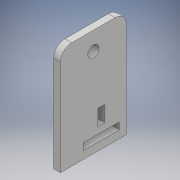
# Autodesk Inventor part: muñeca4
Saved by Autodesk Inventor 2018 (Build 220112000, 112)
## iProperties
Created: 2020-03-11
Part Number: muñeca4
Material: Genérico
Document SubType Name: Modeling
Designer: david
Density: 1 g/cm^3
Appearance: Valor por defecto
Author: david
Autodesk Inventor part; units mm, degrees
ref_plane "YZ Plane" through (0, 0, 0) normal (1, 0, 0) x (0, 1, 0)
ref_plane "XZ Plane" through (0, 0, 0) normal (0, 1, 0) x (-1, 0, 0)
ref_plane "XY Plane" through (0, 0, 0) normal (0, 0, 1) x (1, 0, 0)
sketch "Boceto1" plane through (0, 0, 0) normal (1, 0, 0) x (0, 1, 0)
  line L0 (8, 0) -> (8, -3)
  line L1 (8, -3) -> (-8, -3)
  line L2 (-8, -3) -> (-8, 0)
  line L3 (8, 0) -> (-8, 0)
  line L4 (-18.175, -6.5) -> (11.175, -6.5)
  line L5 (1.5, 3) -> (1.5, 10)
  line L6 (1.5, 10) -> (-1.5, 10)
  line L7 (-1.5, 10) -> (-1.5, 3)
  line L8 (-1.5, 3) -> (1.5, 3)
  line L9 (11.175, -6.5) -> (11.175, 45.5)
  line L10 (-18.175, 45.5) -> (-18.175, -6.5)
  line L11 (6.175, 50.5) -> (1.5, 50.5)
  line L12 (-8.5, 50.5) -> (-13.175, 50.5)
  line L13 (1.5, 50.5) -> (-8.5, 50.5)
  circle A0 centre (-3.5, 33) radius 2.5
  arc A1 (-13.175, 50.5) -> (-18.175, 45.5) centre (-13.175, 45.5) ccw
  arc A2 (11.175, 45.5) -> (6.175, 50.5) centre (6.175, 45.5) ccw
  point P0 (11.175, 50.5)
  point P1 (-18.175, 50.5)
  dimension "d28" = 5
  constraints: 28 end point, 9 perpendicular, 4 point on circle, 4 point on line, 4 tangent, 3 centre point, 2 horizontal, 2 vertical, 1 equal radius
  measures "d28" radius of A1
extrude "Extrusión1" add sketch "Boceto1" along normal blind 3
sketch "Boceto2" plane through (3, 0, 0) normal (1, 0, 0) x (0, 0, -1)
  line L0 (-45.5, -18.175) -> (6.5, -18.175) projected
  line L1 (-41.1093, -18.175) -> (-41.1093, 11.1335)
  line L2 (-41.1093, 11.1335) -> (-52.2815, 13.5312)
  line L3 (-52.2815, 13.5312) -> (-52.6386, -19.4753)
  line L4 (-52.6386, -19.4753) -> (-41.1093, -18.175)
  point P0 (0, 0)
  constraints: 8 end point, 1 point on line, 1 vertical
extrude "Extrusión2" cut sketch "Boceto2" against normal blind 3
fillet "Empalme1" radius 5 2 edges at (1.5, -18.175, 41.1093) (1.5, 11.175, 41.3026)
fillet "Empalme2" radius 5 1 edges at (1.5, 11.1335, 41.1093)
